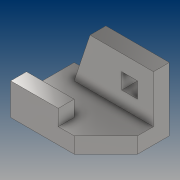
# Autodesk Inventor part: 12
Saved by Autodesk Inventor 2020.2 (Build 242310000, 310)
## iProperties
Created: 2020-09-17
Part Number: 12
Material: 鋼、碳鋼
Document SubType Name: Modeling
Designer: user
Density: 7.85 g/cm^3
Appearance: 半拋光
Mass: 294.375 g
Surface Area: 104.991 cm^2
Volume: 37.5 cm^3
Author: user
Autodesk Inventor part; units mm, degrees
ref_plane "YZ Plane" through (0, 0, 0) normal (1, 0, 0) x (0, 1, 0)
ref_plane "XZ Plane" through (0, 0, 0) normal (0, 1, 0) x (-1, 0, 0)
ref_plane "XY Plane" through (0, 0, 0) normal (0, 0, 1) x (1, 0, 0)
sketch "草圖1" plane through (0, 0, 0) normal (0, 1, 0) x (-1, 0, 0)
  line L0 (0, 0) -> (60, 0)
  line L1 (60, 0) -> (60, 40)
  line L2 (60, 40) -> (0, 40)
  line L3 (0, 40) -> (0, 0)
  line L4 (20, 40) -> (0, 20)
  dimension "d0" = 60
  dimension "d1" = 40
  dimension "d2" = 20
  dimension "d3" = 20
  constraints: 10 end point, 2 parallel, 1 horizontal, 1 midpoint, 1 perpendicular, 1 point on line
  measures "d0" distance of L1.end L2.end
  measures "d1" distance of L0.end L1.end
  measures "d2" distance from line of L0 L4.end
  measures "d3" distance of L2.end L4.start
extrude "擠出1" add sketch "草圖1" along normal blind 10 contours L3 L4 L2 L1 L0
sketch "草圖2" plane through (0, 0, 0) normal (0, 0, -1) x (-1, 0, 0)
  line L0 (0, 0) -> (0, 10) projected
  line L1 (0, 10) -> (60, 10) projected
  line L2 (60, 10) -> (60, 0) projected
  line L3 (60, 0) -> (0, 0) projected
  line L4 (50, 10) -> (40, 40)
  line L5 (40, 40) -> (0, 40)
  line L6 (0, 40) -> (0, 10)
  line L7 (20, 30) -> (10, 30)
  line L8 (10, 30) -> (10, 20)
  line L9 (10, 20) -> (20, 20)
  line L10 (20, 20) -> (20, 30)
  dimension "d6" = 10
  dimension "d7" = 40
  dimension "d8" = 40
  dimension "d9" = 10
  dimension "d10" = 10
  dimension "d11" = 10
  constraints: 14 end point, 3 perpendicular, 2 horizontal, 2 parallel, 1 point on line
  measures "d6" distance from line of L4.start L2
  measures "d7" distance of L4.end L5.end
  measures "d8" distance between parallel lines of L5 L3
  measures "d9" distance of L7.start L7.end
  measures "d10" distance between parallel lines of L6 L8
  measures "d11" distance between parallel lines of L7 L5
extrude "擠出2" add sketch "草圖2" against normal blind 10 contours L6 L5 L4 L1
sketch "草圖3" plane through (0, 10, 0) normal (0, 1, 0) x (1, 0, 0)
  line L0 (-20, -40) -> (-60, -40) projected
  line L1 (-60, -40) -> (-60, 0) projected
  line L2 (-60, 0) -> (-50, 0) projected
  line L3 (-50, -10) -> (-50, 0) projected
  line L4 (0, -10) -> (-50, -10) projected
  line L5 (0, 0) -> (0, -10) projected
  line L6 (-50, 0) -> (0, 0) projected
  line L7 (0, -20) -> (-20, -40) projected
  line L8 (0, -10) -> (0, -20) projected
  line L9 (-60, 0) -> (-60, -40) projected
  line L10 (-60, -40) -> (-30, -40)
  line L11 (-30, -40) -> (-30, -30)
  line L12 (-30, -30) -> (-60, -30)
  line L13 (-60, -30) -> (-60, -40)
  dimension "d14" = 10
  dimension "d15" = 30
  constraints: 8 end point, 2 parallel, 1 horizontal, 1 perpendicular
  measures "d14" distance of L10.end L11.end
  measures "d15" distance of L11.end L12.end
extrude "擠出3" add sketch "草圖3" along normal blind 10 contours L0 L1 L12 L11
